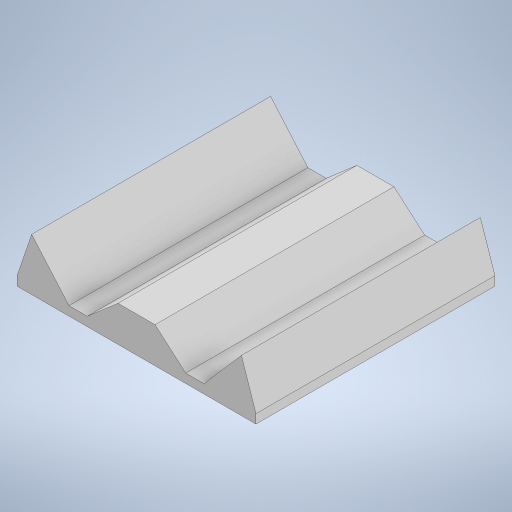
# Autodesk Inventor part: ChargingBase Wstyle - Rough Proto (Flat Bottom)
Saved by Autodesk Inventor 2023 (Build 270158000, 158)
## iProperties
Created: 2022-12-16
Part Number: ChargingBase Wstyle - Rough Proto (Flat Bottom)
Material: Generic
Document SubType Name: Modeling
Designer: ethan
Density: 1 g/cm^3
Appearance: Default
Author: ethan
Autodesk Inventor part; units mm, degrees
ref_plane "YZ Plane" through (0, 0, 0) normal (1, 0, 0) x (0, 1, 0)
ref_plane "XZ Plane" through (0, 0, 0) normal (0, 1, 0) x (-1, 0, 0)
ref_plane "XY Plane" through (0, 0, 0) normal (0, 0, 1) x (1, 0, 0)
sketch "Sketch1" plane through (0, 0, 0) normal (0, 0, 1) x (1, 0, 0)
  line L0 (-228.6, -34.708) -> (-401.2946, 165.1)
  line L1 (-228.6, -34.708) -> (-70.8914, 101.6)
  line L2 (70.8914, 101.6) -> (228.6, -34.708)
  line L3 (228.6, -34.708) -> (401.2946, 165.1)
  line L4 (-70.8914, 101.6) -> (70.8914, 101.6)
  line L5 (0, 0) -> (-457.2, 0) construction
  line L6 (0, 0) -> (457.2, 0) construction
  line L7 (-457.2, 0) -> (-401.2946, 165.1)
  line L8 (457.2, 0) -> (401.2946, 165.1)
  line L9 (-457.2, 0) -> (457.2, 0)
  line L10 (457.2, 0) -> (457.2, -34.708)
  line L11 (457.2, -34.708) -> (-457.2, -34.708)
  line L12 (-457.2, -34.708) -> (-457.2, 0)
  point P0 (258.5982, 0)
  point P1 (188.4428, 0)
  point P2 (-188.4428, 0)
  point P3 (-258.5982, 0)
  dimension "d0" = 90
  dimension "d1" = 90
  dimension "d2" = 141.7828
  dimension "d3" = 101.6
  dimension "d4" = 330.4032
  dimension "d5" = 330.4032
  dimension "d6" = 165.1
  dimension "d7" = 165.1
  dimension "d10" = 70.8914
  dimension "d12" = 457.2
  dimension "d13" = 228.6
  dimension "d14" = 914.4
  constraints: 26 end point, 4 horizontal, 2 parallel, 1 perpendicular
  measures "d0" angle of L1 L0
  measures "d1" angle of L3 L2
  measures "d2" distance of L1.end L2.start
  measures "d3" distance from line of L5.start L4
  measures "d4" horizontal distance of L0.end L1.end
  measures "d5" horizontal distance of L3.end L2.start
  measures "d6" vertical distance of L5.start L3.end
  measures "d7" vertical distance of L0.end L5.start
  measures "d10" horizontal distance of L5.start L1.end
  measures "d12" distance of L2.end L0.start
  measures "d13" horizontal distance of L0.start L5.start
  measures "d14" distance of L6.end L5.end
extrude "Extrusion1" add sketch "Sketch1" along normal blind 914.4
equation "\"d5\" = d4"
equation "\"d6\" = d7"
equation "\"d10\" = 0.5 * d2"
equation "\"d13\" = 0.5 * d12"
body "Solid1"
